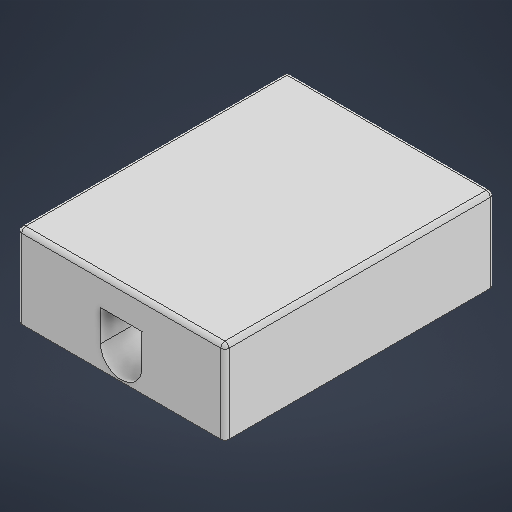
# Autodesk Inventor part: componente
Saved by Autodesk Inventor 2026.2 (Build 302298000, 298)
## iProperties
Created: 2026-01-05
Part Number: componente
Material: Genérico
Document SubType Name: Modeling
Designer: vicho
Density: 1 g/cm^3
Appearance: Valor por defecto
Author: vicho
Autodesk Inventor part; units mm, degrees
ref_plane "YZ Plane" through (0, 0, 0) normal (1, 0, 0) x (0, 1, 0)
ref_plane "XZ Plane" through (0, 0, 0) normal (0, 1, 0) x (-1, 0, 0)
ref_plane "XY Plane" through (0, 0, 0) normal (0, 0, 1) x (1, 0, 0)
sketch "Boceto1" plane through (0, 0, 0) normal (0, 0, 1) x (1, 0, 0)
  line L0 (25, -32.5) -> (-25, -32.5)
  line L1 (-25, -32.5) -> (-25, 32.5)
  line L2 (-25, 32.5) -> (25, 32.5)
  line L3 (25, 32.5) -> (25, -32.5)
  line L4 (25, -32.5) -> (-25, 32.5) construction
  line L5 (-25, -32.5) -> (25, 32.5) construction
  point P0 (0, 0)
  dimension "d0" = 50
  dimension "d1" = 65
  constraints: 12 end point, 2 midpoint, 2 parallel, 1 horizontal, 1 perpendicular
  measures "d0" distance between parallel lines of L3 L1
  measures "d1" distance between parallel lines of L0 L2
extrude "Extrusión1" add sketch "Boceto1" along normal blind 20
sketch "Boceto2" plane through (-25, -32.5, 0) normal (0, -1, 0) x (1, 0, 0)
  line L0 (0, 0) -> (0, 20) projected
  line L1 (0, 13) -> (49.9794, 13)
  line L2 (0, 20) -> (50, 20) projected
  line L3 (0, 28.5169) -> (0, -2.5169) construction
  line L4 (20, 13) -> (20, 5.4006)
  line L5 (30, 13) -> (30, 5.4006)
  line L6 (25, 0) -> (25, 28.5169) construction
  arc A0 (20, 5.4006) -> (30, 5.4006) centre (25, 5.4006) ccw
  point P0 (0, 13)
  dimension "d4" = 7
  dimension "d5" = 10
  dimension "d6" = 49.9794
  dimension "d7" = 14.5994
  dimension "d8" = 8.5169
  dimension "d9" = 8.5169
  constraints: 10 end point, 5 vertical, 4 point on line, 2 point on circle, 2 tangent, 1 centre point, 1 horizontal, 1 midpoint, 1 other
  measures "d4" distance between parallel lines of L2 L1
  measures "d5" distance between parallel lines of L5 L4
  measures "d6" distance from line of L1.end L0
  measures "d7" distance from line of L5.end L2
  measures "d8" distance from line of L6.end L2
  measures "d9" distance from line of L3.start L2
extrude "Extrusión2" cut sketch "Boceto2" against normal blind 15
fillet "Empalme1" radius 1 8 edges at (25, 0, 20) (0, 32.5, 20) (25, 32.5, 10) (-25, 0, 20) (-25, 32.5, 10) (0, -32.5, 20) (-25, -32.5, 10) (25, -32.5, 10)
